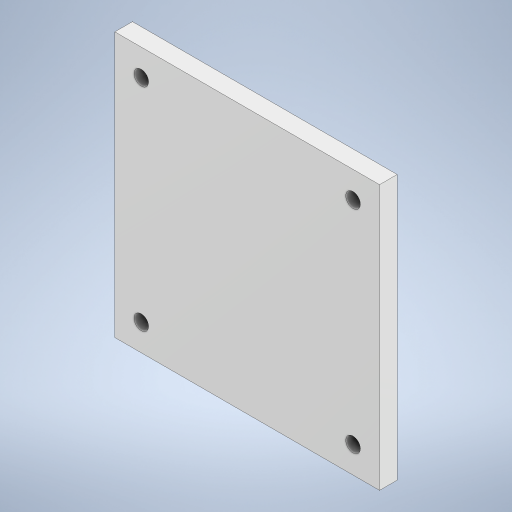
# Autodesk Inventor part: antenna_socket_cap
Saved by Autodesk Inventor 2023 (Build 270158000, 158)
## iProperties
Created: 2023-09-07
Part Number: antenna_socket_cap
Material: Acetal Resin, White
Document SubType Name: Modeling
Designer: 310611102
Density: 1.425 g/cm^3
Appearance: Smooth - White
Mass: 20.325 g
Surface Area: 82.5745 cm^2
Volume: 14.2632 cm^3
Author: 310611102
Autodesk Inventor part; units mm, degrees
ref_plane "YZ Plane" through (0, 0, 0) normal (1, 0, 0) x (0, 1, 0)
ref_plane "XZ Plane" through (0, 0, 0) normal (0, 1, 0) x (-1, 0, 0)
ref_plane "XY Plane" through (0, 0, 0) normal (0, 0, 1) x (1, 0, 0)
sketch "Sketch1" plane through (0, 0, 0) normal (0, 0, 1) x (1, 0, 0)
  line L0 (-30, 30) -> (30, 30)
  line L1 (30, 30) -> (30, -30)
  line L2 (30, -30) -> (-30, -30)
  line L3 (-30, -30) -> (-30, 30)
  line L4 (-30, 30) -> (30, -30) construction
  line L5 (30, 30) -> (-30, -30) construction
  circle A0 centre (-24, 24) radius 1.65
  circle A1 centre (-24, -24) radius 1.65
  circle A2 centre (24, -24) radius 1.65
  circle A3 centre (24, 24) radius 1.65
  point P0 (0, 0)
  dimension "d0" = 60
  dimension "d1" = 60
  dimension "d2" = 3.3
  dimension "d3" = 24
  dimension "d6" = 360
  constraints: 12 end point, 4 centre point, 2 midpoint, 2 parallel, 1 horizontal, 1 perpendicular, 1 point on line, 9 other
  measures "d0" distance of L0.start L0.end
  measures "d1" distance of L0.end L1.end
  measures "d2" diameter of A0
  measures "d3" horizontal distance of point (0, 0) A0.centre
extrude "Extrusion1" add sketch "Sketch1" along normal blind 4
body "Solid1"
